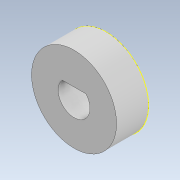
# Autodesk Inventor part: motorbase_5
Saved by Autodesk Inventor 2022 (Build 260153000, 153)
## iProperties
Created: 2023-04-20
Part Number: motorbase_5
Material: 一般
Document SubType Name: Modeling
Designer: JOU
Density: 1 g/cm^3
Appearance: 預設
Author: JOU
Autodesk Inventor part; units mm, degrees
ref_plane "YZ Plane" through (0, 0, 0) normal (1, 0, 0) x (0, 1, 0)
ref_plane "XZ Plane" through (0, 0, 0) normal (0, 1, 0) x (-1, 0, 0)
ref_plane "XY Plane" through (0, 0, 0) normal (0, 0, 1) x (1, 0, 0)
sketch "草圖1" plane through (0, 0, 0) normal (0, 0, 1) x (1, 0, 0)
  circle A0 centre (0, 0) radius 4
  arc A1 (-1.118, 1) -> (1.118, 1) centre (0, 0) ccw
  line L0 (-1.118, 1) -> (1.118, 1)
  line L1 (-1.5, 11.7081) -> (1.5, 11.7081)
  line L2 (1.5, 11.7081) -> (1.5, 3.7081)
  line L3 (1.5, 3.7081) -> (-1.5, 3.7081)
  line L4 (-1.5, 3.7081) -> (-1.5, 11.7081)
  line L5 (-1.5, -3.7081) -> (1.5, -3.7081)
  line L6 (1.5, -3.7081) -> (1.5, -7.7081)
  line L7 (1.5, -7.7081) -> (-1.5, -7.7081)
  line L8 (-1.5, -7.7081) -> (-1.5, -3.7081)
  point P0 (1.5, -3.7081)
  dimension "d0" = 8
  dimension "d1" = 3
  dimension "d2" = 8
  dimension "d3" = 4
  constraints: 18 end point, 5 point on circle, 4 parallel, 2 centre point, 2 collinear, 2 horizontal, 2 perpendicular, 1 coincident
  measures "d0" diameter of A0
  measures "d1" distance of L1.start L1.end
  measures "d2" distance of L1.end L2.end
  measures "d3" distance of L5.end L6.end
extrude "擠出1" add sketch "草圖1" along normal blind 3 contours A0 L5 L3 | L3 A0 | A0 L5
sketch "草圖2" plane through (0, 0, 0) normal (0, 0, -1) x (-1, 0, 0)
  point P0 (0, 0)
sketch "草圖3" plane through (0, 0, 0) normal (0, 0, -1) x (-1, 0, 0)
  circle A0 centre (0, 0) radius 4 projected
  line L0 (1.118, 1) -> (-1.118, 1) projected
  arc A1 (-1.118, 1) -> (1.118, 1) centre (0, 0) ccw projected
